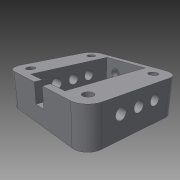
# Autodesk Inventor part: dht22_case_bottom
Saved by Autodesk Inventor 2014 (Build 180170000, 170)
## iProperties
Created: 2016-01-31
Part Number: dht22_case_bottom
Material: Generic
Document SubType Name: Modeling
Designer: buben
Density: 1 g/cm^3
Appearance: Default
Author: buben
Autodesk Inventor part; units mm, degrees
ref_plane "YZ Plane" through (0, 0, 0) normal (1, 0, 0) x (0, 1, 0)
ref_plane "XZ Plane" through (0, 0, 0) normal (0, 1, 0) x (-1, 0, 0)
ref_plane "XY Plane" through (0, 0, 0) normal (0, 0, 1) x (1, 0, 0)
sketch "Sketch1" plane through (0, 0, 0) normal (0, 1, 0) x (-1, 0, 0)
  line L0 (0, 0) -> (-47, 0)
  line L1 (-47, 0) -> (-47, -43)
  line L2 (-47, -43) -> (0, -43)
  line L3 (0, -43) -> (0, 0)
  line L4 (-13, -40) -> (-34, -40) construction
  line L5 (-34, -40) -> (-34, -3) construction
  line L6 (-34, -3) -> (-13, -3) construction
  line L7 (-13, -3) -> (-13, -40) construction
  point P0 (-23.5, -40)
  point P1 (-23.5, -43)
  point P2 (-13, -21.5)
  point P3 (0, -21.5)
  dimension "d2" = 21
  dimension "d3" = 37
  dimension "d11" = 13
  dimension "d12" = 3
  constraints: 16 end point, 4 midpoint, 4 parallel, 2 horizontal, 2 perpendicular, 1 horizontal alignment, 1 vertical alignment
  measures "d2" distance of L4.start L4.end
  measures "d3" distance of L6.end L4.start
  measures "d11" distance between parallel lines of L7 L3
  measures "d12" distance between parallel lines of L4 L2
extrude "Extrusion1" add sketch "Sketch1" along normal blind 3
sketch "Sketch2" plane through (0, 3, 0) normal (0, 1, 0) x (1, 0, 0)
  line L0 (0, 0) -> (47, 0) projected
  line L1 (47, 0) -> (47, 43) projected
  line L2 (47, 43) -> (0, 43) projected
  line L3 (0, 43) -> (0, 0) projected
  line L4 (13, 40) -> (34, 40)
  line L5 (34, 40) -> (34, 3)
  line L6 (34, 3) -> (13, 3)
  line L7 (13, 3) -> (13, 40)
  point P0 (13, 21.5)
  point P1 (0, 21.5)
  point P2 (23.5, 40)
  point P3 (23.5, 43)
  dimension "d15" = 37
  dimension "d16" = 21
  constraints: 8 end point, 4 midpoint, 2 parallel, 1 horizontal, 1 horizontal alignment, 1 perpendicular, 1 vertical alignment
  measures "d15" distance of L6.end L4.start
  measures "d16" distance of L4.start L4.end
extrude "Extrusion2" add sketch "Sketch2" along normal blind 12
sketch "Sketch4" plane through (0, 15, 0) normal (0, 1, 0) x (1, 0, 0)
  line L0 (34, 3) -> (13, 3) projected
  line L1 (0, 0) -> (47, 0) projected
  line L2 (26, 3) -> (21, 3)
  line L3 (21, 3) -> (21, 0)
  line L4 (21, 0) -> (26, 0)
  line L5 (26, 0) -> (26, 3)
  point P0 (23.5, 3)
  point P1 (23.5, 3)
  dimension "d19" = 5
  constraints: 8 end point, 2 midpoint, 2 parallel, 2 point on line, 1 coincident, 1 horizontal, 1 perpendicular
  measures "d19" distance between parallel lines of L5 L3
extrude "Extrusion3" cut sketch "Sketch4" against normal blind 8
sketch "Sketch5" plane through (0, 15, 0) normal (0, 1, 0) x (1, 0, 0)
  line L0 (47, 43) -> (0, 43) projected
  line L1 (0, 43) -> (0, 0) projected
  line L2 (6.5, 36.5) -> (40.5, 36.5) construction
  line L3 (40.5, 36.5) -> (40.5, 6.5) construction
  line L4 (40.5, 6.5) -> (6.5, 6.5) construction
  line L5 (6.5, 6.5) -> (6.5, 36.5) construction
  point P0 (6.5, 21.5)
  point P1 (0, 21.5)
  point P2 (23.5, 36.5)
  point P3 (23.5, 43)
  dimension "d22" = 6.5
  dimension "d23" = 6.5
  constraints: 8 end point, 4 coincident, 4 midpoint, 2 parallel, 1 horizontal, 1 horizontal alignment, 1 perpendicular, 1 vertical alignment
  measures "d22" distance between parallel lines of L1 L5
  measures "d23" distance between parallel lines of L0 L2
hole "Hole1" at (6.5, 15, -36.5) at (6.5, 15, -6.5) at (40.5, 15, -6.5) at (40.5, 15, -36.5) direction (0, -1, 0) diameter 4 end through all
sketch "Sketch7" plane through (47, 0, 0) normal (1, 0, 0) x (0, 0, -1)
  line L0 (0, 0) -> (0, 15)
  circle A0 centre (21.6469, 9) radius 2.25
  circle A1 centre (29.6469, 9) radius 2.25
  circle A2 centre (13.6469, 9) radius 2.25
  dimension "d42" = 4.5
  dimension "d43" = 8
  dimension "d44" = 8
  dimension "d54" = 15
  dimension "d55" = 9
  constraints: 3 centre point, 2 end point, 2 equal radius, 2 horizontal alignment
  measures "d42" diameter of A0
  measures "d43" distance of A0.centre A2.centre
  measures "d44" distance of A1.centre A0.centre
  measures "d54" distance of L0.start L0.end
  measures "d55" vertical distance of L0.start A2.centre
extrude "Extrusion5" cut sketch "Sketch7" against normal through all
sketch "Sketch8" plane through (47, 0, -43) normal (0, 0, -1) x (-1, 0, 0)
  line L0 (0, 0) -> (47, 0) projected
  line L1 (0, 15) -> (47, 15) projected
  line L2 (23.5, 15) -> (23.5, 0) construction
  circle A0 centre (18.5, 9) radius 2.25
  circle A1 centre (28.5, 9) radius 2.25
  dimension "d47" = 4.5
  dimension "d48" = 4.5
  dimension "d49" = 5
  dimension "d50" = 5
  dimension "d56" = 15
  dimension "d57" = 9
  constraints: 2 centre point, 2 end point, 2 midpoint, 1 horizontal alignment
  measures "d47" diameter of A1
  measures "d48" diameter of A0
  measures "d49" distance from line of A0.centre L2
  measures "d50" distance from line of L2 A1.centre
  measures "d56" distance of L0.start L1.start
  measures "d57" vertical distance of L0.start A0.centre
extrude "Extrusion6" cut sketch "Sketch8" against normal up to next
fillet "Fillet2" radius 6 4 edges at (0, 7.5, 0) (47, 7.5, 0) (47, 7.5, -43) (0, 7.5, -43)
sketch "Sketch9" plane through (0, 0, 0) normal (0, -1, 0) x (1, 0, 0)
  circle A0 centre (40.5, -6.5) radius 2 projected
  circle A1 centre (6.5, -36.5) radius 2 projected
  circle A2 centre (6.5, -6.5) radius 2 projected
  circle A3 centre (40.5, -36.5) radius 2 projected
  line L0 (6.5, -10.5415) -> (3, -8.5207)
  line L1 (3, -8.5207) -> (3, -4.4793)
  line L2 (3, -4.4793) -> (6.5, -2.4585)
  line L3 (6.5, -2.4585) -> (10, -4.4793)
  line L4 (10, -4.4793) -> (10, -8.5207)
  line L5 (10, -8.5207) -> (6.5, -10.5415)
  line L6 (10, -38.5207) -> (6.5, -40.5415)
  line L7 (6.5, -40.5415) -> (3, -38.5207)
  line L8 (3, -38.5207) -> (3, -34.4793)
  line L9 (3, -34.4793) -> (6.5, -32.4585)
  line L10 (6.5, -32.4585) -> (10, -34.4793)
  line L11 (10, -34.4793) -> (10, -38.5207)
  line L12 (37, -38.5207) -> (37, -34.4793)
  line L13 (37, -34.4793) -> (40.5, -32.4585)
  line L14 (40.5, -32.4585) -> (44, -34.4793)
  line L15 (44, -34.4793) -> (44, -38.5207)
  line L16 (44, -38.5207) -> (40.5, -40.5415)
  line L17 (40.5, -40.5415) -> (37, -38.5207)
  line L18 (37, -8.5207) -> (37, -4.4793)
  line L19 (37, -4.4793) -> (40.5, -2.4585)
  line L20 (40.5, -2.4585) -> (44, -4.4793)
  line L21 (44, -4.4793) -> (44, -8.5207)
  line L22 (44, -8.5207) -> (40.5, -10.5415)
  line L23 (40.5, -10.5415) -> (37, -8.5207)
  point P0 (0, 0)
  dimension "d58" = 7
  constraints: 48 end point, 4 coincident, 4 vertical, 3 equal length, 52 other
  measures "d58" distance between parallel lines of L0 L3
extrude "Extrusion7" cut sketch "Sketch9" against normal blind 6
equation "\"d23\" = d22"
equation "\"d44\" = d43"
equation "\"d48\" = d47"
equation "\"d50\" = d49"
body "Solid1"
